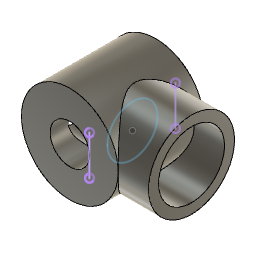
End_Cap_Pivot v1 (Autodesk Fusion 360 design; units mm, degrees)
Autodesk Fusion 360 part; units mm, degrees
sketch "Sketch1" plane through (0, 0, 0) normal (0, 1, 0) x (1, 0, 0)
  circle A0 centre (0, 0) radius 2.75
  circle A1 centre (0, 0) radius 6.75
  dimension "d1" = 5.5
  dimension "d2" = 4
  constraint coincident A0.centre A1.centre
  measures "d1" diameter of A0
extrude "Extrude1" add sketch "Sketch1" along normal blind 12
ref_plane "WorkPlane1" through (3, 0, 0) normal (1, 0, 0) x (0, 1, 0)
sketch "Sketch2" plane through (3, 0, 0) normal (1, 0, 0) x (0, 1, 0)
  line L0 (12, -6.75) -> (12, 6.75)
  line L1 (0, -6.75) -> (0, 6.75)
  circle A0 centre (6, 0) radius 4.6
  circle A1 centre (6, 0) radius 6
  dimension "d6" = 9.2
  dimension "d7" = 6
  dimension "d8" = 12
  dimension "d9" = 1.4
  measures "d6" diameter of A0
  measures "d7" distance of L1 A0.centre
  measures "d8" distance of L0.end L1.end
extrude "Extrude2" add sketch "Sketch2" along normal blind 8
ref_plane "WorkPlane2" through (2.75, 6.403, 0) normal (-1, 0, 0) x (0, 0, -1)
sketch "Sketch3" plane through (2.75, 6.403, 0) normal (-1, 0, 0) x (0, -1, 0)
  line L0 (-5.597, -2.75) -> (-5.597, 2.75)
  line L1 (6.403, -2.75) -> (6.403, 2.75)
  line L2 (6.403, -2.75) -> (6.403, 2.75)
  line L3 (-5.597, -2.75) -> (-5.597, 2.75)
  circle A0 centre (0.403, 0) radius 3.5
  point P0 (0.403, 0)
  dimension "d13" = 6
  dimension "d14" = 12
  dimension "d20" = 7
  constraint coincident P0 A0.centre
  measures "d13" distance of P0 L2
  measures "d14" distance of L1.start L3
  measures "d20" diameter of A0
hole "Hole1" at (2.75, 6, 0) direction (1, 0, 0) diameter 3 depth 10 tip angle 118 counterbore diameter 7 counterbore depth 2
extrude "Extrude3" cut sketch "Sketch3" along normal blind 14.5
equation "d1 = 5 mm + 0.5 mm"
equation "d6 = 9 mm + 0.2 mm"
equation "d7 = d8 / 2"
equation "d13 = d14 / 2"
